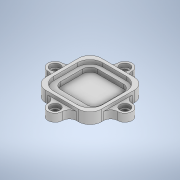
# Autodesk Inventor part: 로드셀 케이스
Saved by Autodesk Inventor 2021 (Build 250183000, 183)
## iProperties
Created: 2021-08-08
Part Number: 로드셀 케이스
Material: 일반
Document SubType Name: Modeling
Designer: Dongyoon
Density: 1 g/cm^3
Appearance: 기본값
Author: Dongyoon
Autodesk Inventor part; units mm, degrees
ref_plane "YZ Plane" through (0, 0, 0) normal (1, 0, 0) x (0, 1, 0)
ref_plane "XZ Plane" through (0, 0, 0) normal (0, 1, 0) x (-1, 0, 0)
ref_plane "XY Plane" through (0, 0, 0) normal (0, 0, 1) x (1, 0, 0)
sketch "스케치1" plane through (0, 0, 0) normal (0, 1, 0) x (-1, 0, 0)
  line L0 (19.5, -19.5) -> (-19.5, -19.5)
  line L1 (-19.5, -19.5) -> (-19.5, 19.5)
  line L2 (-19.5, 19.5) -> (19.5, 19.5)
  line L3 (19.5, 19.5) -> (19.5, -19.5)
  line L4 (19.5, -19.5) -> (-19.5, 19.5) construction
  line L5 (-19.5, -19.5) -> (19.5, 19.5) construction
  point P0 (0, 0)
  dimension "d0" = 39
  dimension "d1" = 39
  constraints: 12 end point, 2 midpoint, 2 parallel, 1 horizontal, 1 perpendicular
  measures "d0" distance of L0.start L0.end
  measures "d1" distance of L0.end L1.end
extrude "돌출1" add sketch "스케치1" along normal blind 5
sketch "스케치2" plane through (0, 5, 0) normal (0, 1, 0) x (1, 0, 0)
  line L0 (-8.25, 17.25) -> (8.25, 17.25)
  line L1 (17.25, 8.25) -> (17.25, -8.25)
  line L2 (8.25, -17.25) -> (-8.25, -17.25)
  line L3 (-17.25, -8.25) -> (-17.25, 8.25)
  line L4 (-17.25, 17.25) -> (17.25, -17.25) construction
  line L5 (17.25, 17.25) -> (-17.25, -17.25) construction
  line L6 (-19.5, -19.5) -> (19.5, -19.5) projected
  line L7 (-19.5, 19.5) -> (19.5, 19.5)
  line L8 (19.5, 19.5) -> (19.5, -19.5)
  line L9 (19.5, -19.5) -> (-19.5, -19.5)
  line L10 (-19.5, -19.5) -> (-19.5, 19.5)
  line L11 (-19.5, 19.5) -> (19.5, -19.5) construction
  line L12 (19.5, 19.5) -> (-19.5, -19.5) construction
  arc A0 (-8.25, 17.25) -> (-17.25, 8.25) centre (-8.25, 8.25) ccw
  arc A1 (17.25, 8.25) -> (8.25, 17.25) centre (8.25, 8.25) ccw
  arc A2 (8.25, -17.25) -> (17.25, -8.25) centre (8.25, -8.25) ccw
  arc A3 (-17.25, -8.25) -> (-8.25, -17.25) centre (-8.25, -8.25) ccw
  point P0 (0, 0)
  dimension "d4" = 34.5
  dimension "d5" = 34.5
  dimension "d6" = 9
  constraints: 24 end point, 8 point on circle, 8 point on line, 8 tangent, 4 centre point, 4 midpoint, 4 parallel, 3 equal radius, 2 horizontal, 2 perpendicular
  measures "d4" distance between parallel lines of L1 L3
  measures "d5" distance between parallel lines of L2 L0
  measures "d6" radius of A0
extrude "돌출2" add sketch "스케치2" along normal blind 2.7
sketch "스케치3" plane through (0, 5, 0) normal (0, 1, 0) x (1, 0, 0)
  line L0 (-14.25, 9.25) -> (-14.25, -6.25)
  line L1 (-9.25, -11.25) -> (9.25, -11.25)
  line L2 (14.25, -6.25) -> (14.25, 9.25)
  line L3 (9.25, 14.25) -> (-9.25, 14.25)
  line L4 (-8.25, 17.25) -> (8.25, 17.25) projected
  line L5 (-17.25, -8.25) -> (-17.25, 8.25) projected
  line L6 (17.25, 8.25) -> (17.25, -8.25) projected
  line L7 (8.25, -17.25) -> (-8.25, -17.25) projected
  arc A0 (-9.25, 14.25) -> (-14.25, 9.25) centre (-9.25, 9.25) ccw
  arc A1 (14.25, 9.25) -> (9.25, 14.25) centre (9.25, 9.25) ccw
  arc A2 (9.25, -11.25) -> (14.25, -6.25) centre (9.25, -6.25) ccw
  arc A3 (-14.25, -6.25) -> (-9.25, -11.25) centre (-9.25, -6.25) ccw
  point P0 (0, 0)
  dimension "d9" = 3
  dimension "d10" = 3
  dimension "d11" = 3
  dimension "d12" = 6
  dimension "d13" = 5
  constraints: 8 end point, 8 point on circle, 8 tangent, 4 centre point, 3 equal radius, 3 perpendicular, 1 vertical
  measures "d9" distance between parallel lines of L4 L3
  measures "d10" distance between parallel lines of L5 L0
  measures "d11" distance between parallel lines of L6 L2
  measures "d12" distance between parallel lines of L7 L1
  measures "d13" radius of A0
extrude "돌출3" cut sketch "스케치3" against normal blind 3
sketch "스케치14" plane through (0, 0, 0) normal (0, 1, 0) x (-1, 0, 0)
  line L0 (-19.5, -19.5) -> (19.5, -19.5) projected
  line L1 (-5, -19.5) -> (5, -19.5)
  line L2 (5, -19.5) -> (5, -29.5)
  line L3 (5, -29.5) -> (-5, -29.5)
  line L4 (-5, -29.5) -> (-5, -19.5)
  line L5 (19.5, 19.5) -> (-19.5, 19.5) projected
  line L6 (5, 19.5) -> (-5, 19.5)
  line L7 (-5, 19.5) -> (-5, 29.5)
  line L8 (-5, 29.5) -> (5, 29.5)
  line L9 (5, 29.5) -> (5, 19.5)
  line L10 (-19.5, 19.5) -> (-19.5, -19.5) projected
  line L11 (-19.5, 5) -> (-29.5, 5)
  line L12 (-29.5, 5) -> (-29.5, -5)
  line L13 (-29.5, -5) -> (-19.5, -5)
  line L14 (-19.5, -5) -> (-19.5, 5)
  line L15 (19.5, -19.5) -> (19.5, 19.5) projected
  line L16 (19.5, -19.5) -> (19.5, 19.5) projected
  line L17 (19.5, 5) -> (29.5, 5)
  line L18 (29.5, 5) -> (29.5, -5)
  line L19 (29.5, -5) -> (19.5, -5)
  line L20 (19.5, -5) -> (19.5, 5)
  point P0 (0, 0)
  dimension "d49" = 10
  dimension "d50" = 5
  dimension "d51" = 10
  dimension "d54" = 10
  dimension "d57" = 10
  dimension "d58" = 10
  dimension "d59" = 5
  dimension "d60" = 10
  dimension "d61" = 10
  dimension "d62" = 10
  dimension "d63" = 5
  constraints: 32 end point, 8 parallel, 5 point on line, 4 horizontal, 4 perpendicular
  measures "d49" distance of L2.end L3.end
  measures "d50" distance from line of point (0, 0) L4
  measures "d51" distance of L7.end L8.end
  measures "d54" distance of L1.end L2.end
  measures "d57" distance of L18.end L19.end
  measures "d58" distance of L17.end L18.end
  measures "d59" distance from line of point (0, 0) L19
  measures "d60" distance of L6.end L7.end
  measures "d61" distance of L11.end L12.end
  measures "d62" distance of L11.start L11.end
  measures "d63" distance from line of point (0, 0) L11
extrude "돌출12" add sketch "스케치14" along normal blind 5.5 contours L0 L2 L3 L4 | L13 L12 L11 L10 | L15 L17 L18 L19 | L7 L8 L9 L5
sketch "스케치17" plane through (0, 5.5, 0) normal (0, 1, 0) x (1, 0, 0)
  circle A0 centre (-24.5, 0) radius 1.95
  circle A1 centre (0, -24.5) radius 1.95
  circle A2 centre (24.5, 0) radius 1.95
  circle A3 centre (0, 24.5) radius 1.95
  line L0 (-19.5, 19.5) -> (-19.5, -19.5) projected
  line L1 (-19.5, 5) -> (-29.5, 5) projected
  line L2 (19.5, 19.5) -> (-19.5, 19.5) projected
  line L3 (5, 19.5) -> (5, 29.5) projected
  line L4 (19.5, -19.5) -> (19.5, 19.5) projected
  line L5 (19.5, -5) -> (29.5, -5) projected
  line L6 (-5, -19.5) -> (-5, -29.5) projected
  line L7 (-5, -29.5) -> (5, -29.5) projected
  point P0 (0, 0)
  dimension "d78" = 3.9
  dimension "d79" = 3.9
  dimension "d80" = 3.9
  dimension "d81" = 3.9
  dimension "d101" = 5
  dimension "d102" = 5
  dimension "d103" = 5
  dimension "d104" = 5
  dimension "d105" = 5
  dimension "d106" = 5
  dimension "d107" = 5
  dimension "d108" = 5
  constraints: 4 centre point
  measures "d78" diameter of A0
  measures "d79" diameter of A3
  measures "d80" diameter of A2
  measures "d81" diameter of A1
  measures "d101" distance from line of A0.centre L0
  measures "d102" distance from line of L1 A0.centre
  measures "d103" distance from line of L2 A3.centre
  measures "d104" distance from line of L3 A3.centre
  measures "d105" distance from line of L4 A2.centre
  measures "d106" distance from line of L5 A2.centre
  measures "d107" distance from line of L6 A1.centre
  measures "d108" distance from line of L7 A1.centre
extrude "돌출15" cut sketch "스케치17" against normal through all
fillet "모깎기1" radius 5 8 edges at (-5, 2.75, 29.5) (5, 2.75, 29.5) (-29.5, 2.75, 5) (-29.5, 2.75, -5) (-5, 2.75, -29.5) (5, 2.75, -29.5) (29.5, 2.75, -5) (29.5, 2.75, 5)
fillet "모깎기2" radius 8 4 edges at (-19.5, 3.85, 19.5) (19.5, 3.85, 19.5) (19.5, 3.85, -19.5) (-19.5, 3.85, -19.5)
fillet "모깎기3" radius 5 8 edges at (-19.5, 2.75, 5) (-5, 2.75, 19.5) (5, 2.75, 19.5) (19.5, 2.75, 5) (-19.5, 2.75, -5) (-5, 2.75, -19.5) (5, 2.75, -19.5) (19.5, 2.75, -5)
sketch "스케치20" plane through (0, 5.5, 0) normal (0, 1, 0) x (1, 0, 0)
  circle A0 centre (-24.5, 0) radius 3.5
  circle A1 centre (0, -24.5) radius 3.5
  circle A2 centre (24.5, 0) radius 3.5
  circle A3 centre (0, 24.5) radius 3.5
  point P0 (0, 0)
  dimension "d95" = 7
  dimension "d96" = 7
  dimension "d97" = 7
  dimension "d98" = 7
  constraints: 4 centre point, 4 coincident
  measures "d95" diameter of A0
  measures "d96" diameter of A1
  measures "d97" diameter of A2
  measures "d98" diameter of A3
extrude "돌출18" cut sketch "스케치20" against normal blind 2.5
